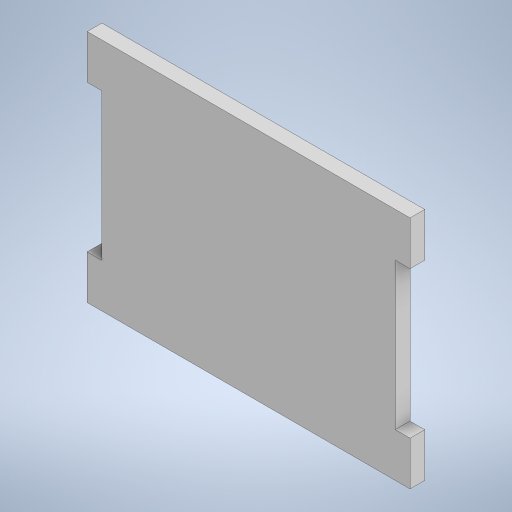
# Autodesk Inventor part: bottomside
Saved by Autodesk Inventor 2024 (Build 280153000, 153)
## iProperties
Created: 2024-04-16
Part Number: bottomside
Material: Generic
Document SubType Name: Modeling
Designer: srika
Density: 1 g/cm^3
Appearance: Default
Author: srika
Autodesk Inventor part; units mm, degrees
ref_plane "YZ Plane" through (0, 0, 0) normal (1, 0, 0) x (0, 1, 0)
ref_plane "XZ Plane" through (0, 0, 0) normal (0, 1, 0) x (-1, 0, 0)
ref_plane "XY Plane" through (0, 0, 0) normal (0, 0, 1) x (1, 0, 0)
sketch "Sketch1" plane through (0, 0, 0) normal (0, 0, 1) x (1, 0, 0)
  line L0 (5, 5) -> (105, 5)
  line L1 (105, 5) -> (105, 85)
  line L2 (105, 85) -> (5, 85)
  line L3 (5, 85) -> (5, 5)
  line L4 (0, 20) -> (5, 20)
  line L5 (5, 20) -> (5, 5)
  line L6 (5, 5) -> (0, 5)
  line L7 (0, 5) -> (0, 20)
  line L8 (0, 85) -> (5, 85)
  line L9 (5, 85) -> (5, 70)
  line L10 (5, 70) -> (0, 70)
  line L11 (0, 70) -> (0, 85)
  line L12 (105, 85) -> (110, 85)
  line L13 (110, 85) -> (110, 70)
  line L14 (110, 70) -> (105, 70)
  line L15 (105, 70) -> (105, 85)
  line L16 (105, 5) -> (110, 5)
  line L17 (110, 5) -> (110, 20)
  line L18 (110, 20) -> (105, 20)
  line L19 (105, 20) -> (105, 5)
  point P0 (0, 0)
  constraints: 40 end point, 10 parallel, 5 horizontal, 5 perpendicular, 5 point on line
extrude "Extrusion1" add sketch "Sketch1" along normal blind 5
body "Solid1"
